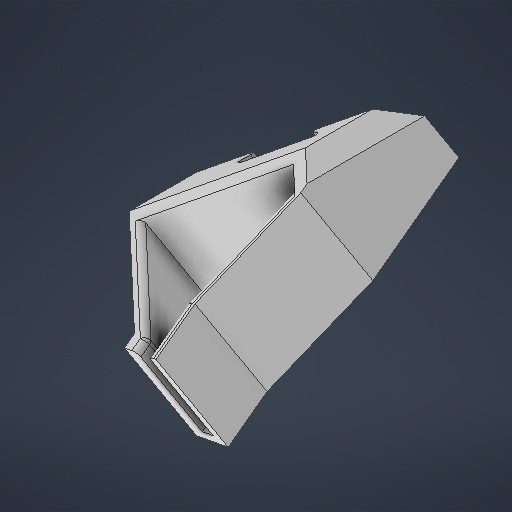
# Autodesk Inventor part: coinDropper
Saved by Autodesk Inventor 2026.1 (Build 301233020, 233B)
## iProperties
Created: 2025-11-01
Part Number: coinDropper
Material: Generic
Document SubType Name: Modeling
Designer: Zain
Density: 1 g/cm^3
Appearance: Default
Author: Zain
Autodesk Inventor part; units mm, degrees
sketch3d "3D Sketch1"
ref_plane "Work Plane1" through (-0.0056, 14.7303, 11.9873) normal (-1, 0, 0) x (0, 0, -1)
ref_plane "Work Plane2" through (-2.9108, 16.1551, 9.4021) normal (-0.7071068, 0.2534044, -0.6601411) x (0.1555934, -0.854939, -0.4948434)
sketch "Sketch2" plane through (-2.9108, 16.1551, 9.4021) normal (-0.7071068, 0.2534044, -0.6601411) x (0.1555934, -0.854939, -0.4948434)
  line L0 (-180, 0) -> (0, 0)
  line L1 (0, 0) -> (0, -32)
  line L2 (0, -32) -> (-180, -32)
  line L3 (-180, -32) -> (-180, 0)
  line L4 (3, -35) -> (-180, -35)
  line L5 (-180, -35) -> (-180, 3)
  line L6 (-180, 3) -> (3, 3)
  line L7 (3, 3) -> (3, -35)
  line L8 (-180, 0.3) -> (0.2, 0.3)
  line L9 (0.2, 0.3) -> (0.2, -32.3)
  line L10 (0.2, -32.3) -> (-180, -32.3)
  line L11 (-180, -32.3) -> (-180, 0.3)
  point P0 (-180, 0)
  dimension "d1" = 180
  dimension "d2" = 32
  dimension "d5" = 3
  dimension "d6" = 3
  dimension "d7" = 3
  dimension "d13" = 0.2
  dimension "d14" = 0.3
  dimension "d15" = 0.3
  constraints: 24 end point, 6 parallel, 3 horizontal, 3 perpendicular, 1 collinear, 1 point on line, 1 other
  measures "d1" distance of L1.end L2.end
  measures "d2" distance of L0.end L1.end
  measures "d5" distance between parallel lines of L2 L4
  measures "d6" distance between parallel lines of L7 L1
  measures "d7" distance between parallel lines of L6 L0
  measures "d13" distance between parallel lines of L9 L1
  measures "d14" distance between parallel lines of L10 L2
  measures "d15" distance between parallel lines of L8 L0
extrude "Extrusion1" add sketch "Sketch2" along normal blind 3
extrude "Extrusion3" add sketch "Sketch2" against normal blind 6 contours L5 L6 L7 L4 L10 L9 L8
ref_plane "Work Plane3" through (19.5768, 30.1922, -13.8415) normal (0, 0, 1) x (1, 0, 0)
sketch "Sketch4" plane through (-3.0866, 15.8483, 9.4727) normal (-0.1555934, 0.854939, 0.4948434) x (0.7071068, -0.2534044, 0.6601411)
  line L0 (0, 0) -> (0, 32.6) projected
  line L1 (0, 0) -> (6, 0) projected
  line L2 (6, 32.6) -> (6, 0) projected
  line L3 (0, 32.6) -> (6, 32.6) projected
  line L4 (5, 32.6) -> (6, 32.0226)
  point P0 (-0.0547, 0.3088)
  dimension "d18" = 5
  dimension "d20" = 30
  constraints: 2 end point, 2 point on line
  measures "d18" distance of L0.end L4.start
  measures "d20" angle of L3 L4
extrude "Extrusion4" [suppressed]
sketch "Sketch5" plane through (19.5768, 30.1922, -13.8415) normal (0, 0, 1) x (1, 0, 0)
  line L0 (-26.2115, -17.1996) -> (-54.6851, 139.2543) projected
  line L1 (-19.8475, -19.4802) -> (-26.2115, -17.1996) projected
  line L2 (-19.8475, -19.4802) -> (6.364, -2.2806) projected
  line L3 (6.364, -2.2806) -> (-22.1096, 154.1732) projected
  line L4 (-54.6851, 139.2543) -> (-28.4736, 156.4538) projected
  line L5 (-28.4736, 156.4538) -> (-22.1096, 154.1732) projected
  point P0 (-19.5768, -30.1922)
extrude "Extrusion5" add sketch "Sketch5" along normal up to next
sketch "Sketch6" plane through (-2.9108, 16.1551, 9.4021) normal (0.7071068, -0.2534044, 0.6601411) x (0.6897758, 0.4526207, -0.5651051)
  line L0 (13.5, 135.3) -> (29, 135.3)
  line L1 (13.5, 109.3) -> (13.5, 135.3)
  line L2 (11.5, 109.3) -> (13.5, 109.3)
  line L3 (11.5, 77.3) -> (11.5, 109.3)
  line L4 (9.5, 77.3) -> (11.5, 77.3)
  line L5 (9.5, 45.3) -> (9.5, 77.3)
  line L6 (6.25, 45.3) -> (9.5, 45.3)
  line L7 (6.25, 2.8) -> (6.25, 45.3)
  line L8 (29, 2.8) -> (6.25, 2.8)
  line L9 (29, 135.3) -> (29, 2.8)
  line L10 (32, 0) -> (32, 180) projected
  line L11 (0, 0) -> (32, 0) projected
  line L12 (32.3, 180) -> (32.3, -0.2) projected
  line L13 (32.3, -0.2) -> (29, -0.2)
  line L14 (29, -0.2) -> (29, 2.8)
  line L15 (29, 2.8) -> (32.3, 2.8)
  line L16 (32.3, 2.8) -> (32.3, -0.2)
  point P0 (0.0088, -18.9171)
  dimension "d25" = 3
  dimension "d26" = 3.3
  constraints: 28 end point, 6 horizontal, 5 vertical, 2 parallel, 1 coincident, 1 perpendicular
  measures "d25" distance of L13.end L14.end
  measures "d26" distance of L14.end L15.end
sketch "Sketch8" plane through (19.5768, 30.1922, -13.8415) normal (0, 0, -1) x (-1, 0, 0)
  line L0 (0.1767, 0.4115) -> (28.2147, 154.4716) projected
  line L1 (50.7014, 139.7161) -> (28.2147, 154.4716) projected
  line L2 (50.7014, 139.7161) -> (22.6634, -14.3439) projected
  line L3 (22.6634, -14.3439) -> (0.1767, 0.4115) projected
  line L4 (18.6122, -8.8144) -> (25.2249, 27.5205) projected
  line L5 (2.9198, 1.4827) -> (18.6122, -8.8144) projected
  line L6 (23.5359, 114.7621) -> (2.9198, 1.4827) projected
  line L7 (25.2249, 27.5205) -> (22.9831, 28.9915) projected
  line L8 (22.9831, 28.9915) -> (27.9621, 56.3496) projected
  line L9 (26.5826, 57.2548) -> (31.5615, 84.6129) projected
  line L10 (27.9621, 56.3496) -> (26.5826, 57.2548) projected
  line L11 (30.182, 85.5181) -> (34.2274, 107.7465) projected
  line L12 (31.5615, 84.6129) -> (30.182, 85.5181) projected
  line L13 (34.2274, 107.7465) -> (23.5359, 114.7621) projected
  line L14 (26.6416, 26.5909) -> (9.5325, 37.8176)
  line L15 (9.5325, 37.8176) -> (7.338, 34.4733)
  line L16 (7.338, 34.4733) -> (24.4471, 23.2466)
  line L17 (24.4471, 23.2466) -> (26.6416, 26.5909)
  line L18 (29.3788, 55.42) -> (27.1843, 52.0757)
  line L19 (27.1843, 52.0757) -> (12.317, 61.8314)
  line L20 (12.317, 61.8314) -> (14.5115, 65.1757)
  line L21 (14.5115, 65.1757) -> (29.3788, 55.42)
  line L22 (32.9782, 83.6833) -> (30.7837, 80.339)
  line L23 (30.7837, 80.339) -> (17.296, 89.1894)
  line L24 (17.296, 89.1894) -> (19.4905, 92.5337)
  line L25 (19.4905, 92.5337) -> (32.9782, 83.6833)
  point P0 (19.5768, -30.1922)
  point P1 (18.7127, 88.2598)
  point P2 (13.7337, 60.9018)
  point P3 (8.7547, 33.5437)
  dimension "d27" = 4
  dimension "d28" = 4
  dimension "d29" = 4
  constraints: 24 end point, 6 parallel, 6 point on line, 3 collinear, 3 perpendicular
  measures "d27" distance between parallel lines of L14 L16
  measures "d28" distance of L19.end L20.end
  measures "d29" distance of L23.end L24.end
extrude "Extrusion6" cut sketch "Sketch8" against normal through all contours L5 L6 L16 L4 | L14 L6 L19 L8 | L6 L23 L9 L21 | L6 L13 L11 L25
ref_plane "Work Plane4" through (-13.5174, 19.9562, -0.5) normal (0.7071068, -0.2534044, 0.6601411) x (0.6897758, 0.4526207, -0.5651051)
ref_plane "Work Plane6" through (-26.4567, 144.2602, 83.7981) normal (-0.1555934, 0.854939, 0.4948434) x (0.7071068, -0.2534044, 0.6601411)
split body "Split1" result two bodies by plane through (-26.4567, 144.2602, 83.7981) normal (-0.1555934, 0.854939, 0.4948434) first body at (-13.9482, 171.37, 41.9041)
split body "Split2" result two bodies by plane through (-13.5174, 19.9562, -0.5) normal (0.7071068, -0.2534044, 0.6601411) bodies 2 first body at (-22.4266, 166.4041, 87.2241)
sketch "Sketch9" plane through (-26.4567, 144.2602, 83.7981) normal (-0.1555934, 0.854939, 0.4948434) x (0.7071068, -0.2534044, 0.6601411)
  line L0 (-15, 7.5724) -> (-15, 45.5724) projected
  line L1 (-13.2929, 19.8653) -> (-11.7071, 18.2796)
  line L2 (-10, 18.9867) -> (-10, 34.1582)
  line L3 (-11.7071, 34.8653) -> (-13.2929, 33.2796)
  arc A0 (-11.7071, 18.2796) -> (-10, 18.9867) centre (-11, 18.9867) ccw
  arc A1 (-10, 34.1582) -> (-11.7071, 34.8653) centre (-11, 34.1582) ccw
  line L4 (-15, 7.5724) -> (-15, 45.5724) projected
  line L5 (-15, 7.5724) -> (-3, -2.7) projected
  line L6 (-3, -2.7) -> (-3, 35.3) projected
  line L7 (-15, 45.5724) -> (-3, 35.3) projected
  line L8 (-15, 45.5724) -> (-15, 53.2768) projected
  line L9 (-15, 45.5724) -> (-3, 35.3) projected
  line L10 (-3, 35.3) -> (6, 35.3) projected
  line L11 (-15, 53.2768) -> (6, 35.3) projected
  line L12 (0, 0) -> (0, 32.6) projected
  line L13 (0, 32.6) -> (6, 32.6) projected
  line L14 (6, 35.3) -> (6, 32.6) projected
  line L15 (-3, 35.3) -> (6, 35.3) projected
  line L16 (-3, -2.7) -> (-3, 35.3) projected
  line L17 (6, -2.7) -> (-3, -2.7) projected
  line L18 (6, 0) -> (6, -2.7) projected
  line L19 (0, 0) -> (6, 0) projected
  line L20 (-15, 45.5724) -> (-15, 53.2768) projected
  line L21 (-34.0212, 69.5596) -> (-15, 53.2768) projected
  line L22 (-15, 33.9867) -> (-15, 53.2768)
  line L23 (-15, 19.1582) -> (-15, 7.5724)
  arc A2 (-13.2929, 19.8653) -> (-15, 19.1582) centre (-14, 19.1582) ccw
  arc A3 (-15, 33.9867) -> (-13.2929, 33.2796) centre (-14, 33.9867) ccw
  line L24 (-15.3, 53.5336) -> (-15.3, 33.9867)
  arc A4 (-15.3, 33.9867) -> (-13.0808, 33.0674) centre (-14, 33.9867) ccw
  line L25 (-13.0808, 33.0674) -> (-11.495, 34.6532)
  arc A5 (-10.3, 34.1582) -> (-11.495, 34.6532) centre (-11, 34.1582) ccw
  line L26 (-10.3, 34.1582) -> (-10.3, 18.9867)
  arc A6 (-11.495, 18.4917) -> (-10.3, 18.9867) centre (-11, 18.9867) ccw
  line L27 (-11.495, 18.4917) -> (-13.0808, 20.0775)
  arc A7 (-13.0808, 20.0775) -> (-15.3, 19.1582) centre (-14, 19.1582) ccw
  line L28 (-15.3, 19.1582) -> (-15.3, 7.8293)
  line L29 (-43.0212, 31.5596) -> (-15, 7.5724) projected
  point P0 (-0.0547, 0.3088)
  point P1 (-15, 21.5724)
  point P2 (-10, 16.5724)
  point P3 (-10, 36.5724)
  point P4 (-15, 31.5724)
  point P5 (-15, 33.9867)
  point P6 (-15, 45.5724)
  point P7 (-15, 33.156)
  point P8 (-15, 19.9889)
  dimension "d35" = 45
  dimension "d36" = 45
  dimension "d37" = 20
  dimension "d38" = 5
  dimension "d40" = 10
  dimension "d41" = 38
  dimension "d42" = 14
  dimension "d47" = 1
  dimension "d48" = 1
  dimension "d49" = 0.3
  constraints: 20 end point, 16 point on circle, 13 point on line, 10 tangent, 8 centre point, 3 vertical, 2 equal radius, 1 collinear, 1 parallel, 6 other
  measures "d35" angle of L2 L1
  measures "d36" angle of L2 L3
  measures "d37" distance of point (-10, 16.572) point (-10, 36.572)
  measures "d38" distance between parallel lines of L2 L0
  measures "d40" distance of point (-15, 31.572) point (-15, 21.572)
  measures "d41" distance of L0.start L0.end
  measures "d42" distance of L0.start point (-15, 21.572)
  measures "d47" radius of A0
  measures "d48" radius of A2
  measures "d49" distance between parallel lines of L2 L26
extrude "Extrusion7" cut sketch "Sketch9" along normal through all contours L29 L28 A7 L0 | L0 A7 L27 A6 L26 A5 L25 A4 A3 L3 A1 L2 A0 L1 A2 | A4 L24 L21 L8 L0 bodies 4 5
sketch "Sketch11" plane through (-26.4567, 144.2602, 83.7981) normal (-0.1555934, 0.854939, 0.4948434) x (0.7071068, -0.2534044, 0.6601411)
  line L0 (34.4958, 0.0029) -> (24.2403, 8.7821)
  line L1 (24.2403, 8.7821) -> (25.6343, 10.4105)
  line L2 (25.6343, 10.4105) -> (35.8898, 1.6314)
  line L3 (35.8898, 1.6314) -> (34.4958, 0.0029)
  line L4 (32.5449, -2.2761) -> (29.886, 0)
  line L5 (29.886, 0) -> (27.5747, -2.7)
  line L6 (27.5747, -2.7) -> (30.2336, -4.9761)
  line L7 (30.2336, -4.9761) -> (32.5449, -2.2761)
  line L8 (34.4958, 0.0029) -> (32.5449, -2.2761)
  line L9 (-11.495, 18.4917) -> (-13.0808, 20.0775) projected
  arc A0 (-15, 19.9889) -> (-15.3, 19.1582) centre (-14, 19.1582) ccw projected
  line L10 (-15, 33.156) -> (-15, 19.9889) projected
  arc A1 (-15.3, 33.9867) -> (-15, 33.156) centre (-14, 33.9867) ccw projected
  line L11 (-13.0808, 33.0674) -> (-11.495, 34.6532) projected
  arc A2 (-10.3, 34.1582) -> (-11.495, 34.6532) centre (-11, 34.1582) ccw projected
  line L12 (-10.3, 34.1582) -> (-10.3, 18.9867) projected
  arc A3 (-11.495, 18.4917) -> (-10.3, 18.9867) centre (-11, 18.9867) ccw projected
  line L13 (6, -2.7) -> (-3, -2.7) projected
  line L14 (-3, -2.7) -> (-43.0212, 31.5596) projected
  line L15 (-15, 7.5724) -> (-15, 19.1582) projected
  arc A4 (-13.2929, 19.8653) -> (-15, 19.1582) centre (-14, 19.1582) ccw projected
  line L16 (-13.2929, 19.8653) -> (-11.7071, 18.2796) projected
  arc A5 (-11.7071, 18.2796) -> (-10, 18.9867) centre (-11, 18.9867) ccw projected
  line L17 (-10, 18.9867) -> (-10, 34.1582) projected
  arc A6 (-10, 34.1582) -> (-11.7071, 34.8653) centre (-11, 34.1582) ccw projected
  line L18 (-11.7071, 34.8653) -> (-13.2929, 33.2796) projected
  arc A7 (-15, 33.9867) -> (-13.2929, 33.2796) centre (-14, 33.9867) ccw projected
  line L19 (-15, 33.9867) -> (-15, 53.2768) projected
  line L20 (-34.0212, 69.5596) -> (6, 35.3) projected
  line L21 (6, 35.3) -> (6, 32.6) projected
  line L22 (6, 32.6) -> (0, 32.6) projected
  line L23 (0, 32.6) -> (0, 0) projected
  line L24 (0, 0) -> (6, 0) projected
  line L25 (6, 0) -> (6, -2.7) projected
  line L26 (-15.3, 19.1582) -> (-15.3, 7.8293) projected
  line L27 (-15.3, 53.5336) -> (-15.3, 33.9867) projected
  line L28 (-3, 35.3) -> (6, 35.3) projected
  line L29 (0, 32.6) -> (6, 32.6) projected
  line L30 (0, 0) -> (0, 32.6) projected
  line L31 (-3, -2.7) -> (-3, 35.3) projected
  line L32 (6, 35.3) -> (6, 32.6) projected
  line L33 (6, -2.7) -> (-3, -2.7) projected
  line L34 (6, 0) -> (6, -2.7) projected
  line L35 (0, 0) -> (6, 0) projected
  line L36 (6, 35.3) -> (6, 32.6) projected
  line L37 (-15.3, 53.5336) -> (6, 35.3) projected
  line L38 (-15, 53.2768) -> (6, 35.3) projected
  line L39 (24.2403, 8.7821) -> (25.905, 10.057)
  line L40 (25.905, 10.057) -> (7.6648, 33.8749)
  line L41 (7.6648, 33.8749) -> (6, 32.6)
  line L42 (6, 32.6) -> (24.2403, 8.7821)
  line L43 (6, 35.3) -> (7.6648, 33.8749)
  line L44 (6, -2.7) -> (27.5747, -2.7)
  line L45 (6, 0) -> (29.886, 0)
  line L46 (24.2403, 8.7821) -> (6, 24.3964) construction
  line L47 (6, 32.6) -> (6, 0) construction
  line L48 (6, 35.3) -> (6, 32.6)
  line L49 (6, 0) -> (6, -2.7) projected
  line L50 (6, 0) -> (6, -2.7)
  line L51 (6, 35.3) -> (6, 32.6) projected
  arc A8 (-13.0808, 20.0775) -> (-15, 19.9889) centre (-14, 19.1582) ccw projected
  arc A9 (-15, 33.156) -> (-13.0808, 33.0674) centre (-14, 33.9867) ccw projected
  line L52 (-15.3, 7.8293) -> (-43.0212, 31.5596) projected
  line L53 (-34.0212, 69.5596) -> (-15.3, 53.5336) projected
  line L54 (-43.0212, 31.5596) -> (-43.0212, 69.5596) projected
  line L55 (-43.0212, 69.5596) -> (-34.0212, 69.5596) projected
  point P0 (-0.0547, 0.3088)
  dimension "d63" = 3
  dimension "d64" = 3.5
  dimension "d65" = 13.5
  dimension "d66" = 30
  dimension "d67" = 24.0107
  constraints: 38 end point, 7 parallel, 4 perpendicular, 3 collinear, 3 point on line, 2 horizontal, 1 vertical
  measures "d63" distance between parallel lines of L4 L0
  measures "d64" distance of L5.end L6.end
  measures "d65" distance of L1.end L2.end
  measures "d66" distance of L21.end L0.end
  measures "d67" distance of L46.end L0.end
extrude "Extrusion8" add sketch "Sketch11" along normal up to surface (30 mm away) contours L0 L39 L40 L2 L3 | L42 L41 L40 L1 | L1 L40 L39 | L7 L6 L5 L4 | L21 L43 L41 | L5 L44 L25 L45 bodies 4
sketch "Sketch12" plane through (-3.97, 159.0156, 65.3757) normal (0.1555934, -0.854939, -0.4948434) x (0.7071068, -0.2534044, 0.6601411)
  arc A0 (-15, 13.4418) -> (-13.2929, 12.7347) centre (-14, 13.4418) ccw projected
  line L0 (-13.2929, 12.7347) -> (-11.7071, 14.3204) projected
  arc A1 (-10, 13.6133) -> (-11.7071, 14.3204) centre (-11, 13.6133) ccw projected
  line L1 (-10, 13.6133) -> (-10, -1.5582) projected
  arc A2 (-11.7071, -2.2653) -> (-10, -1.5582) centre (-11, -1.5582) ccw projected
  line L2 (-11.7071, -2.2653) -> (-13.2929, -0.6796) projected
  arc A3 (-13.2929, -0.6796) -> (-15, -1.3867) centre (-14, -1.3867) ccw projected
  line L3 (-15, -20.6768) -> (-15, -1.3867) projected
  line L4 (-15, -20.6768) -> (7.6648, -1.2749) projected
  line L5 (25.6343, 22.1895) -> (7.6648, -1.2749) projected
  line L6 (35.8898, 30.9686) -> (25.6343, 22.1895) projected
  line L7 (34.4958, 32.5971) -> (35.8898, 30.9686) projected
  line L8 (24.2403, 23.8179) -> (34.4958, 32.5971) projected
  line L9 (6, 0) -> (24.2403, 23.8179) projected
  line L10 (6, 0) -> (0, 0) projected
  line L11 (0, 0) -> (0, 32.6) projected
  line L12 (0, 32.6) -> (29.886, 32.6) projected
  line L13 (32.5449, 34.8761) -> (29.886, 32.6) projected
  line L14 (30.2336, 37.5761) -> (32.5449, 34.8761) projected
  line L15 (27.5747, 35.3) -> (30.2336, 37.5761) projected
  line L16 (27.5747, 35.3) -> (-3, 35.3) projected
  line L17 (-3, 35.3) -> (-15, 25.0276) projected
  line L18 (-15, 13.4418) -> (-15, 25.0276) projected
  line L19 (30.2336, 37.5761) -> (35.8898, 30.9686)
  line L20 (6, 0) -> (6, 32.6)
  point P0 (-0.0547, 32.2912)
  point P1 (34.4958, 32.5971)
  point P2 (32.5449, 34.8761)
  point P3 (34.4958, 32.5971)
  point P4 (32.5449, 34.8761)
  constraints: 4 end point, 2 perpendicular, 1 point on line
extrude "Extrusion9" add sketch "Sketch12" against normal blind 3 contours L19 L8 L9 L20 L12 L13 bodies 4
combine bodies "Combine2" operation type add bodies to combine 5 3
fillet "Fillet1" radius 1.5 7 edges at (-7.3283, 164.4545, 115.5483) (-9.8368, 161.4831, 119.8932) (-20.5582, 166.1217, 108.508) (-7.8914, 150.7934, 111.6921) (-5.8259, 156.199, 103.0022) (-6.1608, 175.442, 96.9323) (-11.4375, 152.6823, 80.0323)
delete faces "Delete Face1" heal no whole lump yes faces at (-24.2286, 169.0466, 72.7125)
delete faces "Delete Face2" heal no whole lump yes faces at (-28.8209, 166.9431, 71.8608)
equation "\"d15\" = d14"
equation "\"d28\" = d27"
equation "\"d29\" = d28"
equation "\"d42\" = -0.5 * d40 + 0.5 * d41"
equation "\"d49\" = doveTailTolerance"
equation "\"doveTailTolerance\" = 0.3"
body "Solid3"
body "Solid4"
